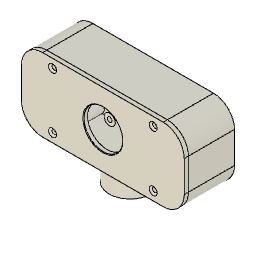
Camera Case (Autodesk Fusion 360 design; units mm, degrees)
Autodesk Fusion 360 part; units mm, degrees
sketch "Board" plane through (0, 0, 0) normal (0, 1, 0) x (1, 0, 0) in component "Camera"
  line L0 (-27, 0) -> (27, 0) construction
  line L1 (0, -11) -> (0, 11) construction
  line L2 (-27, -8) -> (-27, 8)
  line L3 (27, 8) -> (27, -8)
  line L4 (-27, -8) -> (-16, -8)
  line L5 (-27, 8) -> (-16, 8)
  line L6 (27, -8) -> (16, -8)
  line L7 (27, 8) -> (16, 8)
  line L8 (-16, -8) -> (-16, -11)
  line L9 (-16, -11) -> (16, -11)
  line L10 (16, -11) -> (16, -8)
  line L11 (-16, 8) -> (-16, 11)
  line L12 (-16, 11) -> (-6, 11)
  line L13 (16, 8) -> (16, 11)
  line L14 (16, 11) -> (6, 11)
  line L15 (-6, 11) -> (-6, 8)
  line L16 (-6, 8) -> (6, 8)
  line L17 (6, 8) -> (6, 11)
  circle A0 centre (10.05, 8.15) radius 1.15
  circle A1 centre (-10.05, -8.15) radius 1.15
  circle A2 centre (10.175, -8.175) radius 0.825
  circle A3 centre (-10.175, 8.175) radius 0.825
  circle A4 centre (0, 0) radius 6.95
  dimension "d4" = 54
  dimension "d5" = 22
  dimension "d6" = 16
  dimension "d7" = 16
  dimension "d9" = 11
  dimension "d10" = 11
  dimension "d11" = 11
  dimension "d12" = 11
  dimension "d14" = 10
  dimension "d15" = 10
  dimension "d20" = 2.3
  dimension "d23" = 16.95
  dimension "d24" = 2.85
  dimension "d25" = 2.3
  dimension "d26" = 16.95
  dimension "d27" = 2.85
  dimension "d28" = 1.65
  dimension "d29" = 2.825
  dimension "d30" = 1.65
  dimension "d33" = 16.825
  dimension "d34" = 2.825
  dimension "d35" = 16.825
  dimension "d37" = 13.9
  constraint horizontal L0
  constraint midpoint A4.centre L0
  constraint vertical L1
  constraint midpoint A4.centre L1
  constraint vertical L2
  constraint midpoint L0.start L2
  constraint perpendicular L0 L3
  constraint midpoint L0.end L3
  constraint perpendicular L2 L4
  constraint perpendicular L2 L5
  constraint perpendicular L3 L6
  constraint perpendicular L3 L7
  constraint perpendicular L4 L8
  constraint perpendicular L8 L9
  constraint perpendicular L9 L10
  constraint midpoint L1.start L9
  constraint perpendicular L5 L11
  constraint perpendicular L11 L12
  constraint perpendicular L7 L13
  constraint perpendicular L13 L14
  constraint perpendicular L12 L15
  constraint perpendicular L1 L16
  constraint perpendicular L16 L17
  constraint coincident L1.end L12
  constraint coincident L1.end L14
  constraint collinear L5 L16
  constraint coincident A4.centre origin
  measures "d4" distance of L0.start L0.end
  measures "d5" distance of L1.start L1.end
  measures "d6" distance of L2.start L2.end
  measures "d7" distance of L3.start L3.end
  measures "d9" distance of L2.start L4.end
  measures "d10" distance of L2.end L5.end
  measures "d11" distance of L3.end L6.end
  measures "d12" distance of L3.start L7.end
  measures "d14" distance of L11.end L12.end
  measures "d15" distance of L13.end L14.end
  measures "d20" diameter of A0
  measures "d23" distance of L3 A0.centre
  measures "d24" distance of L14 A0.centre
  measures "d25" diameter of A1
  measures "d26" distance of L2 A1.centre
  measures "d27" distance of L9 A1.centre
  measures "d28" diameter of A2
  measures "d29" distance of L9 A2.centre
  measures "d30" diameter of A3
  measures "d33" distance of L3 A2.centre
  measures "d34" distance of L12 A3.centre
  measures "d35" distance of L2 A3.centre
  measures "d37" diameter of A4
sketch "Case" plane through (0, 0, 0) normal (0, 1, 0) x (1, 0, 0) in component "Camera Case Back"
  line L0 (-16, -11) -> (16, -11)
  line L1 (-27, -8) -> (-16, -8)
  line L2 (-16, -8) -> (-16, -11)
  line L3 (-27, -8) -> (-27, 8)
  line L4 (-27, 8) -> (-16, 8)
  line L5 (-16, 11) -> (-6, 11)
  line L6 (-16, 8) -> (-16, 11)
  line L7 (-6, 11) -> (-6, 8)
  line L8 (-6, 8) -> (6, 8)
  line L9 (6, 8) -> (6, 11)
  line L10 (16, 11) -> (6, 11)
  line L11 (16, 8) -> (16, 11)
  line L12 (27, 8) -> (16, 8)
  line L13 (27, 8) -> (27, -8)
  line L14 (27, -8) -> (16, -8)
  line L15 (16, -11) -> (16, -8)
  circle A0 centre (10.175, -8.175) radius 0.825
  circle A1 centre (-10.05, -8.15) radius 1.15
  circle A2 centre (-10.175, 8.175) radius 0.825
  circle A3 centre (10.05, 8.15) radius 1.15
  line L16 (-21.6, -11.6) -> (21.6, -11.6)
  line L17 (27.6, -5.6) -> (27.6, 5.6)
  line L18 (21.6, 11.6) -> (-21.6, 11.6)
  line L19 (-27.6, 5.6) -> (-27.6, -5.6)
  arc A4 (-27.6, -5.6) -> (-21.6, -11.6) centre (-21.6, -5.6) ccw
  arc A5 (-21.6, 11.6) -> (-27.6, 5.6) centre (-21.6, 5.6) ccw
  arc A6 (27.6, 5.6) -> (21.6, 11.6) centre (21.6, 5.6) ccw
  arc A7 (21.6, -11.6) -> (27.6, -5.6) centre (21.6, -5.6) ccw
  circle A8 centre (-10.05, -8.15) radius 2
  circle A9 centre (-10.05, -8.15) radius 0.825
  circle A10 centre (10.175, -8.175) radius 2
  circle A11 centre (10.175, -8.175) radius 0.825
  circle A12 centre (-10.175, 8.175) radius 2
  circle A13 centre (-10.175, 8.175) radius 0.825
  circle A14 centre (10.05, 8.15) radius 2
  circle A15 centre (10.05, 8.15) radius 0.825
  circle A16 centre (18, 10) radius 2
  circle A17 centre (18, 10) radius 0.825
  circle A18 centre (-18, 10) radius 2
  circle A19 centre (-18, -10) radius 2
  circle A20 centre (-18, -10) radius 0.825
  circle A21 centre (18, -10) radius 2
  circle A22 centre (-18, 10) radius 0.825
  circle A23 centre (18, -10) radius 0.825
  line L20 (29.1, -5.6) -> (29.1, 5.6)
  arc A24 (29.1, 5.6) -> (21.6, 13.1) centre (21.6, 5.6) ccw
  line L21 (21.6, 13.1) -> (-21.6, 13.1)
  arc A25 (-21.6, 13.1) -> (-29.1, 5.6) centre (-21.6, 5.6) ccw
  line L22 (-29.1, 5.6) -> (-29.1, -5.6)
  arc A26 (-29.1, -5.6) -> (-21.6, -13.1) centre (-21.6, -5.6) ccw
  line L23 (-21.6, -13.1) -> (21.6, -13.1)
  arc A27 (21.6, -13.1) -> (29.1, -5.6) centre (21.6, -5.6) ccw
  dimension "d39" = 0.6
  dimension "d40" = 0.6
  dimension "d41" = 0.6
  dimension "d42" = 0.6
  dimension "d44" = 6
  dimension "d47" = 4
  dimension "d48" = 1.65
  dimension "d49" = 4
  dimension "d50" = 1.65
  dimension "d51" = 4
  dimension "d52" = 1.65
  dimension "d53" = 4
  dimension "d54" = 1.65
  dimension "d55" = 4
  dimension "d56" = 1.65
  dimension "d57" = 4
  dimension "d58" = 4
  dimension "d59" = 1.65
  dimension "d60" = 4
  dimension "d61" = 1.65
  dimension "d62" = 1.65
  dimension "d64" = 1.5
  constraint horizontal L16
  constraint vertical L17
  constraint horizontal L18
  constraint vertical L19
  constraint tangent L16 A4
  constraint tangent L19 A4
  constraint tangent L18 A5
  constraint tangent L19 A5
  constraint equal A4 A5
  constraint tangent L17 A6
  constraint tangent L18 A6
  constraint equal A4 A6
  constraint tangent L16 A7
  constraint tangent L17 A7
  constraint equal A4 A7
  constraint concentric A1 A8
  constraint concentric A8 A9
  constraint concentric A0 A10
  constraint concentric A0 A11
  constraint concentric A2 A12
  constraint concentric A2 A13
  constraint concentric A3 A14
  constraint concentric A14 A15
  constraint tangent L12 A16
  constraint tangent L11 A16
  constraint concentric A16 A17
  constraint tangent L4 A18
  constraint tangent L6 A18
  constraint concentric A19 A20
  constraint tangent L2 A19
  constraint tangent L15 A21
  constraint concentric A18 A22
  constraint concentric A21 A23
  constraint tangent L1 A19
  constraint tangent L14 A21
  measures "d39" distance of L3 L19
  measures "d40" distance of L13 L17
  measures "d41" distance of L0 L16
  measures "d42" distance of L10 L18
  measures "d44" radius of A4
  measures "d47" diameter of A8
  measures "d48" diameter of A9
  measures "d49" diameter of A10
  measures "d50" diameter of A11
  measures "d51" diameter of A12
  measures "d52" diameter of A13
  measures "d53" diameter of A14
  measures "d54" diameter of A15
  measures "d55" diameter of A16
  measures "d56" diameter of A17
  measures "d57" diameter of A18
  measures "d58" diameter of A19
  measures "d59" diameter of A20
  measures "d60" diameter of A21
  measures "d61" diameter of A22
  measures "d62" diameter of A23
extrude "Extrude1" add sketch "Case" along normal blind 1.5 contours L0 L1 L2 L3 L4 L5 L6 L7 L8 L9 L10 L11 L12 L13 L14 L15 | L0 L2 L15 L16 A19 A21 | L1 L2 A19 | L16 A19 | L14 L15 A21 | L16 A21 | L1 L3 L4 L16 L18 L19 A4 A5 A18 A19 | L16 A19 | L12 L13 L14 L16 L17 L18 A6 A7 A16 A21 | L16 A21 | L4 L6 A18 | L18 A18 | L11 L12 A16 | L18 A16 | L18 A18 | L5 L6 L7 L8 L9 L10 L11 L18 A16 A18 | L18 A16 | A0 A11 | A1 | A2 A13 | A3 | A8 | A9 | A10 | A12 | A14 | A15 | A17 | A20 | A22 | A23 | L20 A24 L21 A25 L22 A26 L23 A27 makes body 1 in component "Camera Case Back"
extrude "Extrude2" add sketch "Case" along normal blind 4 from surface at 1.5 contours A1 | A3 | A8 | A10 | A12 | A14 bodies 1 in component "Camera Case Back"
extrude "Extrude3" add sketch "Case" along normal blind 15 from surface at 1.5 contours L16 A19 | L16 A21 | L16 A19 | L16 A21 | L18 A18 | L18 A16 | L18 A18 | L18 A16 | L20 A24 L21 A25 L22 A26 L23 A27 bodies 1 in component "Camera Case Back"
ref_plane "WorkPlane1" through (0, 8.25, -13.1) normal (0, 0, -1) x (-1, 0, 0) in component "Camera Case Back"
sketch "Socket" plane through (0, 8.25, -13.1) normal (0, 0, -1) x (1, 0, 0) in component "Camera Case Back"
  circle A0 centre (0, 0) radius 7.5
  circle A1 centre (0, 0) radius 6.75
  circle A2 centre (0, 0) radius 0.825
  circle A3 centre (0, 0) radius 2.5
  line L0 (21.6, -8.25) -> (-21.6, -8.25)
  circle A4 centre (7.5, -7.25) radius 2
  line L1 (7.5, 0) -> (7.5, -8.25) construction
  line L2 (7.5, -5.25) -> (14.5, -5.25)
  dimension "d76" = 15
  dimension "d78" = 13.5
  dimension "d81" = 1.65
  dimension "d82" = 5
  dimension "d84" = 4
  dimension "d98" = 3
  constraint coincident A0.centre A1.centre
  constraint coincident A0 L1.start
  constraint coincident L0 L1.end
  constraint perpendicular L0 L1
  constraint tangent A0 L1
  constraint coincident A4.centre L1
  constraint coincident L1 L2.start
  constraint perpendicular L1 L2
  constraint tangent A4 L2
  measures "d76" diameter of A0
  measures "d78" diameter of A1
  measures "d81" diameter of A2
  measures "d82" diameter of A3
  measures "d84" diameter of A4
  measures "d98" distance of L0 L2
extrude "Extrude6" cut sketch "Socket" against normal blind 1.5 contours L0 A4 picked at (6.8813, -7.5434) bodies 1 in component "Camera Case Back"
ref_plane "WorkPlane1" through (0, 16.5, 0) normal (0, 1, 0) x (1, 0, 0) in component "Camera Case Lid"
sketch "Sketch1" plane through (0, 16.5, 0) normal (0, 1, 0) x (1, 0, 0) in component "Camera Case Lid"
  line L0 (-21.6, -13.1) -> (21.6, -13.1)
  arc A0 (21.6, -13.1) -> (29.1, -5.6) centre (21.6, -5.6) ccw
  line L1 (29.1, -5.6) -> (29.1, 5.6)
  arc A1 (29.1, 5.6) -> (21.6, 13.1) centre (21.6, 5.6) ccw
  line L2 (21.6, 13.1) -> (-21.6, 13.1)
  arc A2 (-21.6, 13.1) -> (-29.1, 5.6) centre (-21.6, 5.6) ccw
  line L3 (-29.1, 5.6) -> (-29.1, -5.6)
  arc A3 (-29.1, -5.6) -> (-21.6, -13.1) centre (-21.6, -5.6) ccw
  circle A4 centre (18, -10) radius 0.825
  circle A5 centre (-18, -10) radius 0.825
  circle A6 centre (-18, 10) radius 0.825
  circle A7 centre (18, 10) radius 0.825
  circle A8 centre (0, 0) radius 6.95
extrude "Extrude1'" add sketch "Sketch1" along normal blind 1.5 separate body makes body 2 in component "Camera Case Lid"
chamfer "Chamfer1" distance 0.6 angle 45 4 edges at (17.2308, 18, 9.7017) (17.2308, 18, -10.2983) (-18.7692, 18, -10.2983) (-18.7692, 18, 9.7017) on bodies 2 in component "Camera Case Lid"
chamfer "Chamfer1" distance 0.2 angle 45 1 edges at (-6.4797, 18, -2.5132) on bodies 2 in component "Camera Case Lid"
ref_plane "WorkPlane2" through (0, 8.25, 0) normal (0, 1, 0) x (1, 0, 0) in component "Camera Case Back"
sketch "Sketch6" plane through (0, 8.25, 0) normal (0, 1, 0) x (1, 0, 0) in component "Camera Case Back"
  line L0 (21.6, 13.1) -> (-21.6, 13.1) construction
  line L1 (0, 13.1) -> (0, 37) construction
  line L2 (0, 21.1) -> (7.5, 21.1)
  line L3 (7.5, 21.1) -> (7.5, 13.1)
  line L4 (0, 13.1) -> (7.5, 13.1)
  line L5 (2.5, 21.1) -> (2.5, 13.1)
  line L6 (0.825, 21.1) -> (0.825, 13.1)
  circle A0 centre (0, 25.6) radius 7.5
  point P0 (21.6, 13.1)
  point P1 (-21.6, 13.1)
  point P2 (6, 21.1)
  dimension "d99" = 8
  dimension "d100" = 0.825
  dimension "d101" = 2.5
  dimension "d102" = 7.5
  dimension "d103" = 15
  dimension "d104" = 1.5
  constraint coincident P0 L0.start
  constraint coincident P1 L0.end
  constraint midpoint L0 L1.start
  constraint perpendicular L0 L1
  constraint coincident L1 L2.start
  constraint perpendicular L1 L2
  constraint coincident L0 L3.end
  constraint perpendicular L0 L3
  constraint coincident L2 L5.start
  constraint coincident L0 L5.end
  constraint coincident L2 L6.start
  constraint coincident L0 L6.end
  constraint perpendicular L4 L5
  constraint perpendicular L0 L6
  constraint coincident L1 A0.centre
  constraint coincident A0 P2
  constraint coincident L2 P2
  measures "d99" distance of L2 L4
  measures "d100" distance of L1 L6
  measures "d101" distance of L1 L5
  measures "d102" distance of L1 L3
  measures "d103" diameter of A0
  measures "d104" distance of L3 P2
revolve "Revolve1" add sketch "Sketch6" angle 360 about axis through (0, 8.25, -13.1) along (0, 0, -1) contours L4 L5 L6 A0 | L2 L3 L4 L5 A0 bodies 1 in component "Camera Case Back"
component "Camera" placed x (1, 0, 0) y (0, 1, 0) z (0, 0, 1) at (0, 0, 0)
component "Camera Case Back" placed x (1, 0, 0) y (0, 1, 0) z (0, 0, 1) at (0, 0, 0)
component "Camera Case Lid" placed x (1, 0, 0) y (0, 1, 0) z (0, 0, 1) at (0, 0, 0)
equation "BoardWidth = 54 mm"
equation "BoardHeightMax = 22 mm"
equation "BoardHeightMin = 16 mm"
equation "d4 = BoardWidth"
equation "d5 = BoardHeightMax"
equation "d6 = BoardHeightMin"
equation "d7 = BoardHeightMin"
equation "BoardGroveWidth = 11 mm"
equation "d9 = BoardGroveWidth"
equation "d10 = BoardGroveWidth"
equation "d11 = BoardGroveWidth"
equation "d12 = BoardGroveWidth"
equation "BoardLowerLipWidth = 10 mm"
equation "d14 = BoardLowerLipWidth"
equation "d15 = BoardLowerLipWidth"
equation "BoardBiggerHole = 2.3 mm"
equation "BoardSmallerHole = 1.65 mm"
equation "BoardBiggerHoleDistance1 = 1.7 mm"
equation "BoardBiggerHoleDistance2 = 15.8 mm"
equation "d20 = BoardBiggerHole"
equation "d23 = BoardBiggerHoleDistance2 + BoardBiggerHole / 2"
equation "d24 = BoardBiggerHoleDistance1 + BoardBiggerHole / 2"
equation "d25 = BoardBiggerHole"
equation "d26 = BoardBiggerHoleDistance2 + BoardBiggerHole / 2"
equation "d27 = BoardBiggerHoleDistance1 + BoardBiggerHole / 2"
equation "d28 = BoardSmallerHole"
equation "d29 = BoardSmallerHoleDistance1 + BoardSmallerHole / 2"
equation "d30 = BoardSmallerHole"
equation "BoardSmallerHoleDistance1 = 2 mm"
equation "BoardSmallerHoleDistance2 = 16 mm"
equation "d33 = BoardSmallerHoleDistance2 + BoardSmallerHole / 2"
equation "d34 = BoardSmallerHoleDistance1 + BoardSmallerHole / 2"
equation "d35 = BoardSmallerHoleDistance2 + BoardSmallerHole / 2"
equation "BoardCameraDiameter = 13.9 mm"
equation "d37 = BoardCameraDiameter"
equation "CaseOffset = 0.6 mm"
equation "d39 = CaseOffset"
equation "d40 = CaseOffset"
equation "d41 = CaseOffset"
equation "d42 = CaseOffset"
equation "Fillet = 6 mm"
equation "d44 = Fillet"
equation "OffsetDiameter = 4 mm"
equation "OffsetHoleDiameter = BoardSmallerHole"
equation "d47 = OffsetDiameter"
equation "d48 = OffsetHoleDiameter"
equation "d49 = OffsetDiameter"
equation "d50 = OffsetHoleDiameter"
equation "d51 = OffsetDiameter"
equation "d52 = OffsetHoleDiameter"
equation "d53 = OffsetDiameter"
equation "d54 = OffsetHoleDiameter"
equation "d55 = OffsetDiameter"
equation "d56 = OffsetHoleDiameter"
equation "d57 = OffsetDiameter"
equation "d58 = OffsetDiameter"
equation "d59 = OffsetHoleDiameter"
equation "d60 = OffsetDiameter"
equation "d61 = OffsetHoleDiameter"
equation "d62 = OffsetHoleDiameter"
equation "WallThickness = 1.5 mm"
equation "d64 = WallThickness"
equation "d65 = WallThickness"
equation "BoardBackOffset = 4 mm"
equation "d68 = WallThickness"
equation "d69 = BoardBackOffset"
equation "InnerCaseHeight = 15 mm"
equation "d72 = WallThickness"
equation "d73 = InnerCaseHeight"
equation "d76 = SocketDiameter"
equation "SocketDiameter = 15 mm"
equation "d78 = SocketDiameter - WallThickness"
equation "SocketHoleDiameter = BoardSmallerHole"
equation "SocketInnerDiameter = 5 mm"
equation "d81 = SocketHoleDiameter"
equation "d82 = SocketInnerDiameter"
equation "CableCutoutDiameter = 4 mm"
equation "d84 = CableCutoutDiameter"
equation "SocketHeight = 8 mm"
equation "d91 = -WallThickness"
equation "d94 = WallThickness"
equation "d99 = SocketHeight"
equation "d100 = SocketHoleDiameter / 2"
equation "d101 = SocketInnerDiameter / 2"
equation "d102 = SocketDiameter / 2"
equation "d103 = SocketDiameter"
equation "d104 = WallThickness"
